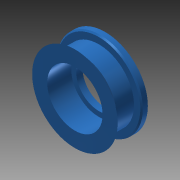
# Autodesk Inventor part: pully 22mmx34mmx10mm
Saved by Autodesk Inventor 2013 (Build 170138000, 138)
## iProperties
Created: 2016-11-25
Part Number: pully 22mmx34mmx10mm
Material: Generic
Document SubType Name: Modeling
Designer: hdv
Density: 1 g/cm^3
Author: hdv
Autodesk Inventor part; units mm, degrees
ref_plane "YZ Plane" through (0, 0, 0) normal (1, 0, 0) x (0, 1, 0)
ref_plane "XZ Plane" through (0, 0, 0) normal (0, 1, 0) x (-1, 0, 0)
ref_plane "XY Plane" through (0, 0, 0) normal (0, 0, 1) x (1, 0, 0)
sketch "Sketch1" plane through (0, 0, 0) normal (0, 0, 1) x (1, 0, 0)
  line L0 (11, 0) -> (17, 0)
  line L1 (17, 0) -> (17, 12) construction
  line L2 (17, 12) -> (11, 12)
  line L3 (11, 12) -> (11, 0)
  line L4 (0, 0) -> (0, 8.5122) construction
  line L5 (14, 9.5) -> (14, 2.5)
  line L6 (14, 9.5) -> (16.5, 9.5)
  line L7 (16.5, 9.5) -> (17, 10)
  line L8 (17, 0) -> (14, 2.5)
  line L9 (17, 10) -> (17, 12)
  line L10 (11, 12) -> (9, 12)
  line L11 (9, 12) -> (9, 9.5)
  line L12 (9, 9.5) -> (11, 9.5)
  line L13 (11, 9.5) -> (11, 12)
  point P0 (17, 0.6699)
  point P1 (17, 6)
  point P2 (15.2143, 7.5754)
  point P3 (15.2143, 2.4246)
  point P4 (14, 6)
  point P5 (17.7886, 0.302)
  point P6 (11, 6)
  dimension "d6" = 12
  dimension "d7" = 11
  dimension "d14" = 6
  dimension "d17" = 7
  dimension "d18" = 2.5
  dimension "d19" = 135
  dimension "d20" = 3
  dimension "d21" = 2
  dimension "d22" = 2.5
  constraints: 28 end point, 4 parallel, 3 midpoint, 3 perpendicular, 2 horizontal, 2 horizontal alignment, 2 point on line, 2 vertical, 1 coincident, 1 collinear
  measures "d6" distance of L1.end L0.end
  measures "d7" distance from line of L3 point (0, 0)
  measures "d14" distance of L0.start L0.end
  measures "d17" distance of L5.start L5.end
  measures "d18" distance of L5.start L6.end
  measures "d19" angle of L7 L6
  measures "d20" distance between parallel lines of L1 L5
  measures "d21" distance of L12.end L11.end
  measures "d22" distance of L11.end L10.end
revolve "Revolution1" add sketch "Sketch1" angle 360 about axis through (0, 0, 0) along (0, 1, 0)
body "Solid1"
